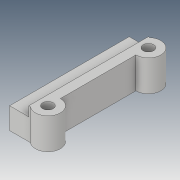
# Autodesk Inventor part: rectSotto
Saved by Autodesk Inventor 2019 (Build 230136000, 136)
## iProperties
Created: 2020-09-16
Part Number: rectSotto
Material: Generic
Document SubType Name: Modeling
Designer: giacomo
Density: 1 g/cm^3
Appearance: Default
Author: giacomo
Autodesk Inventor part; units mm, degrees
ref_plane "YZ Plane" through (0, 0, 0) normal (1, 0, 0) x (0, 1, 0)
ref_plane "XZ Plane" through (0, 0, 0) normal (0, 1, 0) x (-1, 0, 0)
ref_plane "XY Plane" through (0, 0, 0) normal (0, 0, 1) x (1, 0, 0)
sketch "Sketch1" plane through (0, 0, 0) normal (0, 1, 0) x (-1, 0, 0)
  line L0 (4.5194, 15.534) -> (-1.4806, 15.534)
  line L1 (-1.4806, 15.534) -> (-1.4806, -9.466)
  line L2 (-1.4806, -9.466) -> (4.5194, -9.466)
  line L3 (4.5194, -9.466) -> (4.5194, 15.534)
  point P0 (0, 0)
  dimension "d0" = 25
  dimension "d1" = 6
  constraints: 8 end point, 2 parallel, 1 horizontal, 1 perpendicular
  measures "d0" distance of L0.end L1.end
  measures "d1" distance of L1.end L2.end
extrude "Extrusion1" add sketch "Sketch1" along normal blind 4.5
sketch "Sketch2" plane through (0, 4.5, 0) normal (0, 1, 0) x (1, 0, 0)
  line L0 (1.4806, -15.534) -> (1.4806, 9.466) projected
  line L1 (-4.5194, -15.534) -> (1.4806, -15.534) projected
  line L2 (-0.1807, 9.466) -> (-0.5194, 9.466)
  line L3 (-0.5194, 9.466) -> (-0.5194, -15.534)
  line L4 (-0.5194, -15.534) -> (-0.1807, -15.534)
  circle A0 centre (1.4806, 7.466) radius 1.1
  circle A1 centre (1.4806, -13.534) radius 1.1
  arc A2 (-0.1807, -15.534) -> (1.4806, -10.934) centre (1.4806, -13.534) ccw
  arc A3 (1.4806, 4.866) -> (-0.1807, 9.466) centre (1.4806, 7.466) ccw
  line L5 (1.4806, -10.934) -> (1.4806, 4.866)
  point P0 (0, 0)
  point P1 (1.4806, 10.066)
  point P2 (1.4806, -16.134)
  dimension "d4" = 2
  dimension "d5" = 2.2
  dimension "d6" = 0
  dimension "d8" = 2
  dimension "d9" = 2.2
  dimension "d10" = 0
  dimension "d11" = 2
  dimension "d17" = 1.5
  dimension "d18" = 1.5
  constraints: 8 end point, 4 centre point, 4 point on circle, 2 parallel, 2 point on line, 1 horizontal, 1 perpendicular
  measures "d4" distance of L0.end L2.end
  measures "d5" diameter of A0
  measures "d6" distance from line of L0 A0.centre
  measures "d8" distance from line of L2 A0.centre
  measures "d9" diameter of A1
  measures "d10" distance from line of L0 A1.centre
  measures "d11" distance from line of L1 A1.centre
  measures "d17" radial gap between concentric circles of A1 A2
  measures "d18" radial gap between concentric circles of A0 A3
extrude "Extrusion3" add sketch "Sketch2" along normal blind 2 and the other way blind 4.5 contours L0 A1 L1 L3 L2 A3 | A2 L1 L0 A1
extrude "Extrusion4" cut sketch "Sketch2" along normal through all both and the other way through all contours A0 L0 | L0 A0 | A1 L0 | L0 A1
body "Solid1"
